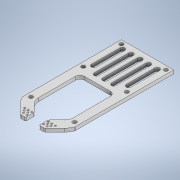
# Autodesk Inventor part: twoSidedHeadplateHolder_wide_sendcutsend
Saved by Autodesk Inventor 2022.1 (Build 261234000, 234)
## iProperties
Created: 2022-07-07
Part Number: twoSidedHeadplateHolder_wide_sendcutsend
Material: Generic
Document SubType Name: Modeling
Designer: Noah
Density: 1 g/cm^3
Appearance: Default
Author: Noah
Autodesk Inventor part; units mm, degrees
ref_plane "YZ Plane" through (0, 0, 0) normal (1, 0, 0) x (0, 1, 0)
ref_plane "XZ Plane" through (0, 0, 0) normal (0, 1, 0) x (-1, 0, 0)
ref_plane "XY Plane" through (0, 0, 0) normal (0, 0, 1) x (1, 0, 0)
sketch "Sketch1" plane through (0, 0, 0) normal (0, 1, 0) x (-1, 0, 0)
  line L0 (-45.1427, 41.275) -> (-45.1427, -0.6244)
  arc A0 (-52.0007, -0.6244) -> (-45.1427, -0.6244) centre (-48.5717, -0.6244) ccw
  line L1 (-52.0007, -0.6244) -> (-52.0007, 41.275)
  arc A1 (-45.1427, 41.275) -> (-52.0007, 41.275) centre (-48.5717, 41.275) ccw
  arc A2 (-26.6007, -0.6244) -> (-23.1717, -4.0534) centre (-23.1717, -0.6244) ccw
  line L2 (-26.6007, -0.6244) -> (-26.6007, 50.1756)
  arc A3 (-23.1717, 53.6046) -> (-26.6007, 50.1756) centre (-23.1717, 50.1756) ccw
  arc A4 (-32.5697, 50.1756) -> (-39.1737, 50.1756) centre (-35.8717, 50.1756) ccw
  line L3 (-32.5697, 50.1756) -> (-32.5697, -0.6244)
  arc A5 (-39.1737, -0.6244) -> (-32.5697, -0.6244) centre (-35.8717, -0.6244) ccw
  line L4 (-39.1737, -0.6244) -> (-39.1737, 50.1756)
  line L5 (-23.1717, 61.3516) -> (-42.2217, 61.3516)
  arc A6 (-48.5717, 67.7016) -> (-42.2217, 61.3516) centre (-42.2217, 67.7016) ccw
  line L6 (-48.5717, 67.7016) -> (-48.5717, 122.1945)
  arc A7 (-44.852, 131.1748) -> (-48.5717, 122.1945) centre (-35.8717, 122.1945) ccw
  line L7 (-44.852, 131.1748) -> (-33.9759, 142.0509)
  arc A8 (-33.9759, 142.0509) -> (-33.046, 144.2959) centre (-36.221, 144.2959) ccw
  line L8 (-33.046, 144.2959) -> (-33.046, 154.7283)
  arc A9 (-33.046, 154.7283) -> (-34.316, 155.9983) centre (-34.316, 154.7283) ccw
  line L9 (-34.316, 155.9983) -> (-36.8109, 155.9983)
  line L10 (-61.2717, 122.3315) -> (-61.2717, -11.8004)
  line L11 (-61.2717, -11.8004) -> (-23.1717, -11.8004)
  circle A10 centre (-35.2685, 151.7756) radius 1.1303 construction
  circle A11 centre (-37.5862, 148.3847) radius 1.1303 construction
  circle A12 centre (-40.3485, 144.9938) radius 1.1303 construction
  circle A13 centre (-40.3485, 151.7756) radius 1.1303 construction
  circle A14 centre (-40.3485, 144.9938) radius 1.1303 construction
  circle A15 centre (-42.6662, 148.3847) radius 1.1303 construction
  circle A16 centre (-45.4285, 144.9938) radius 1.1303 construction
  line L12 (-34.316, 155.9983) -> (-39.3509, 155.9983)
  line L13 (-41.5959, 155.0684) -> (-55.1707, 141.4936)
  line L14 (-61.2717, 122.3315) -> (-61.2717, 131.5606)
  arc A17 (-55.1707, 141.4936) -> (-61.0225, 132.7936) centre (-35.8717, 122.1945) ccw
  arc A18 (-39.3509, 155.9983) -> (-41.5959, 155.0684) centre (-39.3509, 152.8233) ccw
  arc A19 (-61.0225, 132.7936) -> (-61.2717, 131.5606) centre (-58.0967, 131.5606) ccw
  line L15 (-23.1717, 61.3516) -> (-23.1717, 53.6046)
  line L16 (-23.1717, -4.0534) -> (-23.1717, -11.8004)
  circle A20 centre (-35.2685, 144.9938) radius 1.22
  circle A21 centre (-35.2685, 151.7756) radius 1.2192
  circle A22 centre (-37.5862, 148.3847) radius 1.2192
  circle A23 centre (-40.3485, 151.7756) radius 1.2192
  circle A24 centre (-42.6662, 148.3847) radius 1.2192
  circle A25 centre (-40.3485, 144.9938) radius 1.2192
  circle A26 centre (-45.4285, 144.9938) radius 1.2192
  line L17 (-54.9217, 50.1756) -> (-54.9217, 126.3756) construction
  circle A27 centre (-54.9217, 126.3756) radius 2.7813
  circle A28 centre (-54.9217, 50.1756) radius 2.7813
  line L18 (-61.2717, -11.8004) -> (-55.5567, -11.8004)
  line L19 (-55.5567, -11.8004) -> (-55.5567, -6.0854) construction
  line L20 (-55.5567, -6.0854) -> (-61.2717, -6.0854) construction
  line L21 (-61.2717, -6.0854) -> (-61.2717, -11.8004)
  circle A29 centre (-55.5567, -6.0854) radius 2.7813
  point P0 (-41.301, 144.2959)
  point P1 (-41.8909, 152.8233)
  point P2 (-61.2717, 132.1817)
  point P3 (-26.6007, -0.6244)
  point P4 (-32.5697, -0.6244)
  point P5 (-52.0007, -0.6244)
  point P6 (-45.1427, -0.6244)
  dimension "d2" = 3.175
  dimension "d12" = 2.44
  dimension "d13" = 2.4384
  dimension "d14" = 2.4384
  dimension "d15" = 2.4384
  dimension "d16" = 2.4384
  dimension "d17" = 2.4384
  dimension "d18" = 2.4384
  dimension "d19" = 76.2
  dimension "d20" = 5.5626
  dimension "d21" = 5.5626
  dimension "d23" = 5.715
  dimension "d24" = 5.715
  dimension "d25" = 5.5626
  constraints: 44 end point, 30 centre point, 27 point on circle, 10 coincident, 5 tangent, 2 horizontal, 2 parallel, 2 vertical, 1 equal radius, 1 perpendicular, 1 point on line
  measures "d2" radius of A18
  measures "d12" diameter of A20
  measures "d13" diameter of A21
  measures "d14" diameter of A22
  measures "d15" diameter of A23
  measures "d16" diameter of A24
  measures "d17" diameter of A25
  measures "d18" diameter of A26
  measures "d19" distance of L17.start L17.end
  measures "d20" diameter of A27
  measures "d21" diameter of A28
  measures "d23" distance of L20.end L19.end
  measures "d24" distance of L19.end L18.end
  measures "d25" diameter of A29
extrude "Extrusion3" add sketch "Sketch1" along normal blind 5
mirror "Mirror2" about plane through (23.1717, 0, 53.6046) normal (-1, 0, 0)
body "Solid2"
